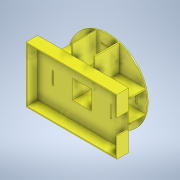
# Autodesk Inventor part: Mass
Saved by Autodesk Inventor 2020 (Build 240168000, 168)
## iProperties
Created: 2022-11-12
Part Number: Mass
Material: PLA
Document SubType Name: Modeling
Designer: Hp
Density: 1.3 g/cm^3
Appearance: Yellow
Author: Hp
## iProperties of the stored document _3DPrint.ipt
Created: 2022-11-12
Part Number: _3DPrint
Material: Generic
Document SubType Name: Modeling
Designer: Hp
Density: 1 g/cm^3
Appearance: Default
Author: Hp
Autodesk Inventor part; units mm, degrees
ref_plane "YZ Plane" through (0, 0, 0) normal (1, 0, 0) x (0, 1, 0)
ref_plane "XZ Plane" through (0, 0, 0) normal (0, 1, 0) x (-1, 0, 0)
ref_plane "XY Plane" through (0, 0, 0) normal (0, 0, 1) x (1, 0, 0)
sketch "Sketch1" plane through (0, 0, 0) normal (0, 0, 1) x (1, 0, 0)
  circle A0 centre (0, 0) radius 37.5
  dimension "d0" = 75
  constraints: 1 centre point, 1 coincident
  measures "d0" diameter of A0
extrude "Extrusion1" add sketch "Sketch1" along normal blind 1
sketch "Sketch2" plane through (0, 0, 1) normal (0, 0, 1) x (1, 0, 0)
  line L0 (-10, -10) -> (10, -10)
  line L1 (10, -10) -> (10, 10)
  line L2 (10, 10) -> (-10, 10)
  line L3 (-10, 10) -> (-10, -10)
  line L4 (-10, 10) -> (10, 10)
  line L5 (10, 10) -> (10, 36.1421)
  line L6 (-10, 36.1421) -> (-10, 10)
  line L7 (10, 10) -> (36.1421, 10)
  line L8 (36.1421, -10) -> (10, -10)
  line L9 (10, -10) -> (10, 10)
  line L10 (-10, -10) -> (10, -10)
  line L11 (10, -10) -> (10, -36.1421)
  line L12 (-10, -36.1421) -> (-10, -10)
  line L13 (-10, -10) -> (-36.1421, -10)
  line L14 (-36.1421, 10) -> (-10, 10)
  line L15 (-10, 10) -> (-10, -10)
  line L16 (35.8504, 11) -> (10, 11)
  line L17 (9, 9) -> (9, -9)
  line L18 (10, -11) -> (35.8504, -11)
  line L19 (11, 10) -> (11, 35.8504)
  line L20 (-11, 35.8504) -> (-11, 10)
  line L21 (-10, 11) -> (-35.8504, 11)
  line L22 (-35.8504, -11) -> (-10, -11)
  line L23 (-9, -9) -> (-9, 9)
  line L24 (-9, -9) -> (9, -9)
  line L25 (11, -10) -> (11, -35.8504)
  line L26 (-11, -35.8504) -> (-11, -10)
  line L27 (-9, 9) -> (9, 9)
  line L28 (9, 9) -> (9, -9)
  line L29 (9, -9) -> (-9, -9)
  line L30 (10, -10) -> (9, -9) construction
  line L31 (-9, 9) -> (-10, 10) construction
  line L32 (-10, -10) -> (-9, -9) construction
  line L33 (9, 9) -> (10, 10) construction
  circle A0 centre (0, 0) radius 37.5
  line L34 (-9, -49.0456) -> (-11, -49.0456)
  point P0 (-11, -11)
  point P1 (11, -11)
  point P2 (-11, 11)
  point P3 (11, 11)
  dimension "d3" = 20
  dimension "d4" = 20
  dimension "d5" = 1
  dimension "d6" = 1
  dimension "d7" = 1
  dimension "d8" = 1
  dimension "d9" = 1
  constraints: 70 end point, 12 parallel, 7 point on line, 5 horizontal, 5 perpendicular, 1 coincident, 18 other
  measures "d3" distance of L2.end L1.end
  measures "d4" distance of L1.end L0.end
  measures "d5" distance between parallel lines of L7 L16
  measures "d6" distance between parallel lines of L5 L19
  measures "d7" distance between parallel lines of L14 L21
  measures "d8" distance between parallel lines of L12 L26
  measures "d9" distance between parallel lines of L2 L27
extrude "Extrusion2" add sketch "Sketch2" along normal blind 23 contours L3 L2 L1 L0 | L12 L22 L26 L13 | L8 L25 L18 L11 | L14 L20 L21 L6 | L12 A0 L26 L22 | L26 L22 A0 L13 | L5 L16 L19 L7 | L8 A0 L18 L25 | L18 L25 A0 L11 | L21 L20 A0 L6 | L14 A0 L21 L20 | L5 A0 L19 L16 | L19 L16 A0 L7
sketch "Sketch5" plane through (0, 0, 1) normal (0, 0, 1) x (1, 0, 0)
  line L0 (10, -10) -> (10, 10) projected
  line L1 (36.1421, -10) -> (10, -10) projected
  line L2 (10, 10) -> (27, 10)
  line L3 (27, 10) -> (27, -10)
  line L4 (27, -10) -> (10, -10)
  line L5 (10, -10) -> (10, 10)
  line L6 (27, 0) -> (27.5, 0)
  line L7 (27, -6) -> (28, -6)
  line L8 (28, -6) -> (28, 6)
  line L9 (28, 6) -> (27, 6)
  line L10 (27, 6) -> (27, -6)
  line L11 (27, -6) -> (28, 6) construction
  line L12 (28, -6) -> (27, 6) construction
  line L13 (-10, 10) -> (-10, -10) projected
  line L14 (-10, 0) -> (-27.5, 0)
  line L15 (-28, -6) -> (-27, -6)
  line L16 (-27, -6) -> (-27, 6)
  line L17 (-27, 6) -> (-28, 6)
  line L18 (-28, 6) -> (-28, -6)
  line L19 (-28, -6) -> (-27, 6) construction
  line L20 (-27, -6) -> (-28, 6) construction
  line L21 (10, -10) -> (-10, -10) projected
  line L22 (0, -10) -> (0, -27.5)
  line L23 (-6, -28) -> (6, -28)
  line L24 (6, -28) -> (6, -27)
  line L25 (6, -27) -> (-6, -27)
  line L26 (-6, -27) -> (-6, -28)
  line L27 (-6, -28) -> (6, -27) construction
  line L28 (6, -28) -> (-6, -27) construction
  line L29 (10, 10) -> (-10, 10) projected
  line L30 (0, 10) -> (0, 27.5)
  line L31 (-6, 27) -> (6, 27)
  line L32 (6, 27) -> (6, 28)
  line L33 (6, 28) -> (-6, 28)
  line L34 (-6, 28) -> (-6, 27)
  line L35 (-6, 27) -> (6, 28) construction
  line L36 (6, 27) -> (-6, 28) construction
  point P0 (0, 0)
  dimension "d21" = 17
  dimension "d22" = 0.5
  dimension "d23" = 1
  dimension "d24" = 12
  dimension "d25" = 17.5
  dimension "d26" = 1
  dimension "d27" = 12
  dimension "d28" = 17.5
  dimension "d29" = 12
  dimension "d30" = 1
  dimension "d31" = 17.5
  dimension "d32" = 12
  dimension "d33" = 1
  constraints: 64 end point, 12 midpoint, 10 parallel, 7 horizontal, 5 perpendicular, 2 vertical, 1 point on line
  measures "d21" distance of L3.end L4.end
  measures "d22" distance of L6.start L6.end
  measures "d23" distance of L9.end L8.end
  measures "d24" distance of L8.end L7.end
  measures "d25" distance of L14.start L14.end
  measures "d26" distance of L17.end L16.end
  measures "d27" distance of L16.end L15.end
  measures "d28" distance of L22.start L22.end
  measures "d29" distance of L25.end L24.end
  measures "d30" distance of L24.end L23.end
  measures "d31" distance of L30.start L30.end
  measures "d32" distance of L33.end L32.end
  measures "d33" distance of L32.end L31.end
extrude "Extrusion5" cut sketch "Sketch5" along normal blind 93 and the other way blind 11.5 contours L25 L24 L23 L26 | L16 L15 L18 L17 | L31 L34 L33 L32 | L3 L9 L8 L7
sketch "Sketch6" plane through (10, -10, 1) normal (1, 0, 0) x (0, 0, -1)
  line L0 (-7.5, 9) -> (-7.5, 11) projected
  line L1 (-7.5, 10) -> (0, 10)
  line L2 (0, 20) -> (0, 0) projected
  line L3 (0, 10) -> (-2, 10)
  line L4 (-3, 14) -> (-1, 14)
  line L5 (-1, 14) -> (-1, 6)
  line L6 (-1, 6) -> (-3, 6)
  line L7 (-3, 6) -> (-3, 14)
  line L8 (-3, 14) -> (-1, 6) construction
  line L9 (-1, 14) -> (-3, 6) construction
  point P0 (1, 10)
  dimension "d36" = 2
  dimension "d37" = 2
  dimension "d38" = 8
  constraints: 16 end point, 4 midpoint, 2 parallel, 1 horizontal, 1 perpendicular, 1 point on line
  measures "d36" distance of L1.end L3.end
  measures "d37" distance of L5.end L6.end
  measures "d38" distance of L4.end L5.end
extrude "Extrusion6" cut sketch "Sketch6" against normal blind 23
sketch "Sketch7" plane through (-10, -10, 1) normal (0, -1, 0) x (1, 0, 0)
  line L0 (11, 7.5) -> (9, 7.5) projected
  line L1 (10, 7.5) -> (10, -0.0458)
  line L2 (10, -0.0458) -> (10, 1.9542)
  line L3 (6, 2.9542) -> (14, 2.9542)
  line L4 (14, 2.9542) -> (14, 0.9542)
  line L5 (14, 0.9542) -> (6, 0.9542)
  line L6 (6, 0.9542) -> (6, 2.9542)
  line L7 (6, 2.9542) -> (14, 0.9542) construction
  line L8 (14, 2.9542) -> (6, 0.9542) construction
  point P0 (10, -1)
  dimension "d41" = 2
  dimension "d42" = 8
  constraints: 16 end point, 3 midpoint, 2 parallel, 1 horizontal, 1 perpendicular, 1 point on line, 1 vertical
  measures "d41" distance of L1.end L2.end
  measures "d42" distance of L4.end L5.end
extrude "Extrusion7" cut sketch "Sketch7" against normal blind 23
sketch "Sketch8" plane through (-10, -10, 1) normal (0, -1, 0) x (1, 0, 0)
  line L0 (6, 0.9542) -> (6, 2.9542) projected
  line L1 (4, 0) -> (16, 0) projected
  line L2 (6, 2.9542) -> (14, 2.9542)
  line L3 (14, 2.9542) -> (14, 0)
  line L4 (14, 0) -> (6, 0)
  line L5 (6, 0) -> (6, 2.9542)
  line L6 (6, 0) -> (14, 0)
  line L7 (14, 0) -> (14, 4)
  line L8 (14, 4) -> (6, 4)
  line L9 (6, 4) -> (6, 0)
  point P0 (10, -1)
  dimension "d45" = 8
  dimension "d46" = 8
  dimension "d47" = 4
  constraints: 16 end point, 4 parallel, 2 horizontal, 2 perpendicular, 1 point on line
  measures "d45" distance of L3.end L4.end
  measures "d46" distance of L8.end L7.end
  measures "d47" distance of L7.end L6.end
extrude "Extrusion8" cut sketch "Sketch8" against normal blind 23
sketch "Sketch9" plane through (10, -10, 1) normal (1, 0, 0) x (0, 0, -1)
  line L0 (-3, 14) -> (-3, 6) projected
  line L1 (-3, 14) -> (0, 14)
  line L2 (0, 14) -> (0, 6)
  line L3 (0, 6) -> (-3, 6)
  line L4 (-3, 6) -> (-3, 14)
  line L5 (0, 6) -> (-4, 6)
  line L6 (-4, 6) -> (-4, 14)
  line L7 (-4, 14) -> (0, 14)
  line L8 (0, 14) -> (0, 6)
  point P0 (1, 10)
  dimension "d50" = 3
  dimension "d51" = 8
  dimension "d52" = 4
  constraints: 16 end point, 4 parallel, 2 horizontal, 2 perpendicular, 1 point on line
  measures "d50" distance of L2.end L3.end
  measures "d51" distance of L1.end L2.end
  measures "d52" distance of L6.end L7.end
extrude "Extrusion9" cut sketch "Sketch9" against normal blind 23
sketch "Sketch10" plane through (0, 0, 24) normal (0, 0, 1) x (1, 0, 0)
  line L0 (42, 25.5) -> (-42, 25.5)
  line L1 (-42, 25.5) -> (-42, -25.5)
  line L2 (-42, -25.5) -> (42, -25.5)
  line L3 (42, -25.5) -> (42, 25.5)
  line L4 (42, 25.5) -> (-42, -25.5) construction
  line L5 (-42, 25.5) -> (42, -25.5) construction
  point P0 (0, 0)
  dimension "d55" = 84
  dimension "d56" = 51
  constraints: 12 end point, 2 midpoint, 2 parallel, 1 horizontal, 1 perpendicular
  measures "d55" distance of L2.end L1.end
  measures "d56" distance of L1.end L0.end
extrude "Extrusion10" add sketch "Sketch10" along normal blind 1
sketch "Sketch11" plane through (0, 0, 25) normal (0, 0, 1) x (1, 0, 0)
  line L0 (11, -25.5) -> (42, -25.5) projected
  line L1 (-42, 25.5) -> (42, 25.5)
  line L2 (42, 25.5) -> (42, -25.5)
  line L3 (42, -25.5) -> (-42, -25.5)
  line L4 (-42, -25.5) -> (-42, 25.5)
  line L5 (-42, 25.5) -> (42, -25.5) construction
  line L6 (42, 25.5) -> (-42, -25.5) construction
  line L7 (43, -26.5) -> (43, 26.5)
  line L8 (43, 26.5) -> (-43, 26.5)
  line L9 (-43, 26.5) -> (-43, -26.5)
  line L10 (-43, -26.5) -> (43, -26.5)
  point P0 (0, 0)
  dimension "d59" = 1
  constraints: 20 end point, 4 parallel, 2 midpoint, 2 perpendicular, 1 horizontal, 3 other
  measures "d59" distance between parallel lines of L2 L7
extrude "Extrusion11" add sketch "Sketch11" along normal blind 10 and the other way blind 1
sketch "Sketch12" plane through (0, 0, 25) normal (0, 0, 1) x (1, 0, 0)
  line L0 (9, -9) -> (-9, -9)
  line L1 (-9, -9) -> (-9, 9)
  line L2 (-9, 9) -> (9, 9)
  line L3 (9, 9) -> (9, -9)
  line L4 (9, -9) -> (-9, 9) construction
  line L5 (-9, -9) -> (9, 9) construction
  point P0 (0, 0)
  dimension "d64" = 18
  dimension "d65" = 18
  constraints: 12 end point, 2 midpoint, 2 parallel, 1 horizontal, 1 perpendicular
  measures "d64" distance of L1.end L2.end
  measures "d65" distance of L0.end L1.end
extrude "Extrusion12" cut sketch "Sketch12" against normal blind 10
sketch "Sketch13" plane through (0, 0, 0) normal (0, 0, -1) x (-1, 0, 0)
  line L0 (-6, 27) -> (6, 27) projected
  line L1 (6, 27) -> (6, 28) projected
  line L2 (-6, 27) -> (6, 27)
  line L3 (6, 27) -> (6, 28)
  line L4 (6, 28) -> (-6, 28)
  line L5 (-6, 28) -> (-6, 27)
  line L6 (-28, -6) -> (-28, 6) projected
  line L7 (-28, 6) -> (-27, 6) projected
  line L8 (-28, -6) -> (-27, -6)
  line L9 (-27, -6) -> (-27, 6)
  line L10 (-27, 6) -> (-28, 6)
  line L11 (-28, 6) -> (-28, -6)
  line L12 (6, -28) -> (6, -27) projected
  line L13 (6, -28) -> (-6, -28)
  line L14 (-6, -28) -> (-6, -27)
  line L15 (-6, -27) -> (6, -27)
  line L16 (6, -27) -> (6, -28)
  line L17 (28, 6) -> (28, -6) projected
  line L18 (27, 6) -> (28, 6) projected
  line L19 (28, -6) -> (27, -6)
  line L20 (27, -6) -> (27, 6)
  line L21 (27, 6) -> (28, 6)
  line L22 (28, 6) -> (28, -6)
  point P0 (0, 0)
  constraints: 32 end point, 8 parallel, 4 horizontal, 4 perpendicular
extrude "Extrusion13" cut sketch "Sketch13" along normal mid plane 93
sketch "Sketch14" plane through (43, -26.5, 35) normal (1, 0, 0) x (0, 0, -1)
  line L0 (11, 16.5) -> (11, 36.5) projected
  line L1 (11, 26.5) -> (0, 26.5)
  line L2 (0, 0) -> (0, 53) projected
  line L3 (21, 34) -> (1, 34)
  line L4 (1, 34) -> (1, 19)
  line L5 (1, 19) -> (21, 19)
  line L6 (21, 19) -> (21, 34)
  line L7 (21, 34) -> (1, 19) construction
  line L8 (1, 34) -> (21, 19) construction
  line L9 (0, 19) -> (10, 19)
  line L10 (10, 19) -> (10, 34)
  line L11 (10, 34) -> (0, 34)
  line L12 (0, 34) -> (0, 19)
  point P0 (35, 26.5)
  dimension "d72" = 20
  dimension "d73" = 15
  dimension "d74" = 10
  constraints: 22 end point, 4 midpoint, 4 parallel, 2 horizontal, 2 perpendicular, 2 point on line
  measures "d72" distance of L5.end L4.end
  measures "d73" distance of L4.end L3.end
  measures "d74" distance of L11.end L10.end
extrude "Extrusion14" cut sketch "Sketch14" against normal blind 3 contours L5 L4 L1 L10 | L1 L4 L3 L10 | L9 L2 L1 L4 | L1 L2 L11 L4
body "Solid1"
